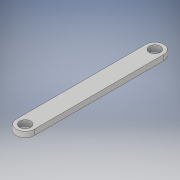
# Autodesk Inventor part: linkage
Saved by Autodesk Inventor 2018 (Build 220112000, 112)
## iProperties
Created: 2018-07-12
Part Number: linkage
Material: Generic
Document SubType Name: Modeling
Designer: Cole Tucker
Density: 1 g/cm^3
Appearance: Default
Author: Cole Tucker
Autodesk Inventor part; units mm, degrees
ref_plane "YZ Plane" through (0, 0, 0) normal (1, 0, 0) x (0, 1, 0)
ref_plane "XZ Plane" through (0, 0, 0) normal (0, 1, 0) x (-1, 0, 0)
ref_plane "XY Plane" through (0, 0, 0) normal (0, 0, 1) x (1, 0, 0)
sketch "Sketch1" plane through (0, 0, 0) normal (0, 1, 0) x (-1, 0, 0)
  line L0 (0, 0) -> (0, -74.3966) construction
  circle A0 centre (0, 0) radius 5.08
  circle A1 centre (0, -74.3966) radius 5.08
  line L1 (5.08, 0) -> (5.08, -74.3966)
  line L2 (-5.08, -74.3966) -> (-5.08, 0)
  dimension "d0" = 74.3966
  dimension "d1" = 10.16
  dimension "d2" = 10.16
  constraints: 6 end point, 4 point on circle, 2 centre point, 2 coincident, 2 tangent, 2 vertical, 1 parallel
  measures "d0" distance of L0.start L0.end
  measures "d1" diameter of A0
  measures "d2" diameter of A1
extrude "Extrusion1" add sketch "Sketch1" along normal blind 3.175
sketch "Sketch2" plane through (0, 3.175, 0) normal (0, 1, 0) x (1, 0, 0)
  arc A0 (5.08, 74.3966) -> (-5.08, 74.3966) centre (0, 74.3966) ccw projected
  point P0 (0, 0)
  point P1 (0, 0)
  constraints: 2 coincident
hole "Hole1" at (0, 3.175, 0) at (0, 3.175, -74.3966) direction (0, -1, 0) diameter 6.35 depth 25.4 tip angle 118
body "Solid1"
